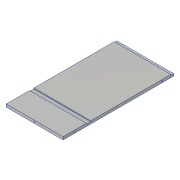
# Autodesk Inventor part: bottom
Saved by Autodesk Inventor 2018 (Build 220112000, 112)
## iProperties
Created: 2015-10-13
Part Number: bottom
Material: Aluminum 6061
Document SubType Name: Modeling
Designer: Sawaiz
Density: 2.7 g/cm^3
Appearance: Aluminum - Flat
Mass: 409.813 g
Surface Area: 530.639 cm^2
Volume: 151.782 cm^3
Author: Sawaiz
Autodesk Inventor part; units mm, degrees
ref_plane "YZ Plane" through (0, 0, 0) normal (1, 0, 0) x (0, 1, 0)
ref_plane "XZ Plane" through (0, 0, 0) normal (0, 1, 0) x (-1, 0, 0)
ref_plane "XY Plane" through (0, 0, 0) normal (0, 0, 1) x (1, 0, 0)
sketch "Sketch1" plane through (0, 0, 0) normal (0, 0, 1) x (1, 0, 0)
  line L0 (-123.7861, -63.5) -> (123.7861, -63.5)
  line L1 (123.7861, -63.5) -> (123.7861, 63.5)
  line L2 (123.7861, 63.5) -> (-123.7861, 63.5)
  line L3 (-123.7861, 63.5) -> (-123.7861, -63.5)
  line L4 (-123.7861, -63.5) -> (123.7861, 63.5) construction
  line L5 (123.7861, -63.5) -> (-123.7861, 63.5) construction
  point P0 (0, 0)
  dimension "d0" = 247.5723
  dimension "d1" = 127
  constraints: 12 end point, 2 midpoint, 2 parallel, 1 horizontal, 1 perpendicular
  measures "d0" distance of L2.end L1.end
  measures "d1" distance of L1.end L0.end
extrude "Extrusion1" add sketch "Sketch1" along normal blind 6.35
sketch "Sketch13" plane through (0, 0, 6.35) normal (0, 0, 1) x (1, 0, 0)
  line L0 (-123.7861, -63.5) -> (123.7861, -63.5) projected
  line L1 (123.7861, -63.5) -> (123.7861, 63.5) projected
  line L2 (123.7861, 63.5) -> (-123.7861, 63.5) projected
  line L3 (-123.7861, 63.5) -> (-123.7861, -63.5) projected
  line L4 (-123.7861, -63.5) -> (123.7861, -63.5) projected
  line L5 (71.7161, -63.5) -> (62.0895, -63.5)
  line L6 (62.0895, -63.5) -> (62.0895, 63.5)
  line L7 (62.0895, 63.5) -> (71.7161, 63.5)
  line L8 (71.7161, 63.5) -> (71.7161, -63.5)
  point P0 (0, 0)
  dimension "d96" = 9.6266
  dimension "d97" = 52.07
  constraints: 8 end point, 2 parallel, 2 point on line, 1 horizontal, 1 perpendicular
  measures "d96" distance between parallel lines of L6 L8
  measures "d97" distance between parallel lines of L1 L8
extrude "Extrusion7" cut sketch "Sketch13" against normal blind 1.6891 contours L6 L2 L8 L0
sketch "Sketch14" plane through (-123.7861, 63.5, 0) normal (0, 1, 0) x (1, 0, 0)
  line L0 (185.8757, -6.35) -> (185.8757, -4.6609) projected
  line L1 (185.8757, -4.6609) -> (195.5023, -4.6609) projected
  line L2 (195.5023, -4.6609) -> (195.5023, -6.35) projected
  line L3 (247.5723, -6.35) -> (195.5023, -6.35) projected
  line L4 (247.5723, 0) -> (247.5723, -6.35) projected
  line L5 (247.5723, 0) -> (0, 0) projected
  line L6 (0, 0) -> (0, -6.35) projected
  line L7 (185.8757, -6.35) -> (0, -6.35) projected
  point P0 (123.7861, 0)
  point P1 (222.1723, -3.175)
  point P2 (25.4, -3.175)
  dimension "d100" = 25.4
  dimension "d101" = 25.4
  dimension "d102" = 3.175
  dimension "d103" = 3.175
  measures "d100" distance from line of L6 point (25.4, -3.175)
  measures "d101" distance from line of L4 point (222.172, -3.175)
  measures "d102" distance from line of L3 point (222.172, -3.175)
  measures "d103" distance from line of L7 point (25.4, -3.175)
hole "Hole6" at (98.3861, 63.5, 3.175) at (-98.3861, 63.5, 3.175) direction (0, -1, 0) diameter 2.156 depth 8.865 tip angle 118 thread size "4-40 UNC" class "2B" standard "ANSI Unified Screw Threads"
mirror "Mirror5" about plane through (0, 0, 0) normal (0, 1, 0) of "Hole6"
sketch "Sketch15" plane through (0, 0, 6.35) normal (0, 0, 1) x (1, 0, 0)
  line L0 (62.0895, -63.5) -> (62.0895, 63.5) projected
  line L1 (62.0895, -63.5) -> (62.0895, 63.5) projected
  line L2 (62.0895, 63.5) -> (-123.7861, 63.5) projected
  line L3 (-123.7861, 63.5) -> (-123.7861, -63.5) projected
  line L4 (-123.7861, -63.5) -> (62.0895, -63.5) projected
  line L5 (-123.7861, -63.5) -> (123.7861, -63.5) projected
  line L6 (123.7861, 63.5) -> (-123.7861, 63.5) projected
  line L7 (-117.3345, -63.5) -> (-123.7861, -63.5)
  line L8 (-123.7861, -63.5) -> (-123.7861, 63.5)
  line L9 (-123.7861, 63.5) -> (-117.3345, 63.5)
  line L10 (-117.3345, 63.5) -> (-117.3345, -63.5)
  point P0 (0, 0)
  dimension "d111" = 185.8757
  dimension "d112" = 6.4516
  constraints: 8 end point, 2 parallel, 2 point on line, 1 horizontal, 1 perpendicular
  measures "d111" distance between parallel lines of L0 L8
  measures "d112" distance between parallel lines of L10 L8
extrude "Extrusion8" cut sketch "Sketch15" against normal blind 1.6891 contours L4 L3 L2 L10
sketch "Sketch16" plane through (123.7861, -63.5, 0) normal (1, 0, 0) x (0, 0, -1)
  line L0 (0, 0) -> (0, 127) projected
  line L1 (0, 127) -> (-6.35, 127) projected
  line L2 (-6.35, 0) -> (-6.35, 127) projected
  line L3 (0, 0) -> (-6.35, 0) projected
  point P0 (0, 63.5)
  point P1 (-3.175, 63.5)
  dimension "d115" = 63.5
  dimension "d116" = 3.175
  measures "d115" distance from line of L3 point (-3.175, 63.5)
  measures "d116" distance from line of L0 point (-3.175, 63.5)
hole "Hole7" at (123.7861, 0, 3.175) direction (-1, 0, 0) diameter 2.156 depth 8.865 tip angle 118 thread size "4-40 UNC" class "2B" standard "ANSI Unified Screw Threads"
equation "\"d0\" = depth"
equation "\"d1\" = width"
equation "\"d2\" = caseThickness"
equation "\"d98\" = alignmentGrooveDepth + alignmentGrooveClearance"
equation "\"d100\" = 4 * caseThickness"
equation "\"d101\" = 4 * caseThickness"
equation "\"d102\" = 0.5 * caseThickness"
equation "\"d103\" = 0.5 * caseThickness"
equation "\"width\" = 127"
equation "\"depth\" = 247.57228"
equation "\"focalLength\" = 185.82488"
equation "\"aerogelHolderDepth\" = 38.24501"
equation "\"caseThickness\" = 6.35"
equation "\"alignmentGrooveDepth\" = 1.5875"
equation "\"alignmentGrooveClearance\" = 0.1016"
equation "\"height\" = 127"
equation "\"mirrorAngle\" = 2.5deg"
equation "\"mirrorThickness\" = 3.175"
equation "\"fresnelThickness\" = 0.254"
equation "\"ior\" = 1.49"
equation "\"centerThickness\" = 1.27"
equation "\"fresnelAngle\" = 90deg"
equation "\"fresnelEffectiveDiameter\" = 152.4"
equation "\"frontPanelThickness\" = 1.5875"
equation "\"fresnelGrooveWidth\" = 9.525"
equation "\"lensDiameter\" = 101.6"
equation "\"lensCenterThickness\" = 16.99999"
equation "\"lensMountThickness\" = 9.525"
equation "\"lensInsetDepth\" = 6.35"
body "Solid1"
